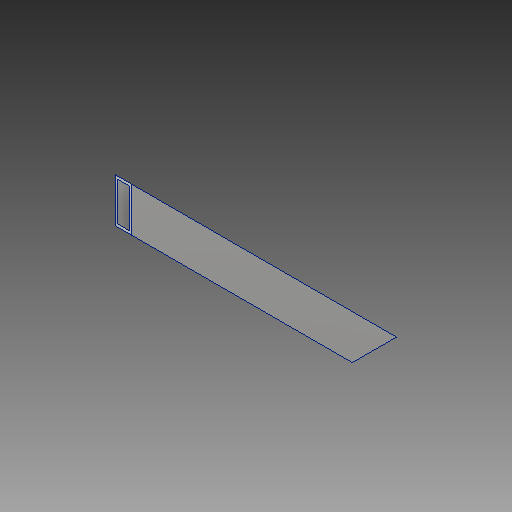
# Autodesk Inventor part: liftanglebar
Saved by Autodesk Inventor 2019 (Build 230136000, 136)
## iProperties
Created: 2019-01-13
Part Number: liftanglebar
Material: Aluminum 6061
Document SubType Name: Modeling
Designer: lebraddock
Density: 2.7 g/cm^3
Appearance: Aluminum - Flat
Mass: 670.473 g
Surface Area: 1576.79 cm^2
Volume: 248.323 cm^3
Author: lebraddock
Autodesk Inventor part; units mm, degrees
ref_plane "YZ Plane" through (0, 0, 0) normal (1, 0, 0) x (0, 1, 0)
ref_plane "XZ Plane" through (0, 0, 0) normal (0, 1, 0) x (-1, 0, 0)
ref_plane "XY Plane" through (0, 0, 0) normal (0, 0, 1) x (1, 0, 0)
sketch "Sketch1" plane through (0, 0, 0) normal (1, 0, 0) x (0, 1, 0)
  line L0 (0, -444.5) -> (444.5, 0)
  line L1 (-35.921, -408.579) -> (408.579, 35.921)
  line L2 (0, -444.5) -> (-35.921, -408.579)
  line L3 (408.579, 35.921) -> (444.5, 0)
  point P0 (0, 0)
  dimension "d1" = 444.5
  dimension "d3" = 50.8
  constraints: 8 end point, 2 parallel
  measures "d1" distance of point (0, 0) L0.start
  measures "d3" distance between parallel lines of L0 L1
extrude "Extrusion1" add sketch "Sketch1" along normal blind 25.4
sketch "Sketch2" plane through (0, 408.579, 35.921) normal (0, 0.7071, 0.7071) x (1, 0, 0)
  line L0 (0, 50.8) -> (0, 0) projected
  line L1 (0, 0) -> (25.4, 0)
  line L2 (25.4, 0) -> (25.4, 50.8)
  line L3 (25.4, 50.8) -> (0, 50.8)
  line L4 (0, 50.8) -> (0, 0)
  line L5 (3.175, 47.625) -> (22.225, 47.625)
  line L6 (22.225, 47.625) -> (22.225, 3.175)
  line L7 (22.225, 3.175) -> (3.175, 3.175)
  line L8 (3.175, 3.175) -> (3.175, 47.625)
  point P0 (0, -263.509)
  dimension "d6" = 3.175
  constraints: 16 end point, 4 parallel, 2 perpendicular, 1 horizontal, 3 other
  measures "d6" distance between parallel lines of L3 L5
extrude "Extrusion2" cut sketch "Sketch2" against normal blind 762 contours L5 L6 L7 L8
sketch "Sketch3" plane through (25.4, 0, 0) normal (1, 0, 0) x (0, 0, -1)
  line L0 (444.5, 0) -> (0, 444.5) projected
  line L1 (0, 444.5) -> (0, 339.9202)
  line L2 (0, 339.9202) -> (302.3662, 0)
  line L3 (302.3662, 0) -> (653.5481, 0)
  line L4 (653.5481, 0) -> (477.9571, -156.1918)
  line L5 (477.9571, -156.1918) -> (43.0071, -156.1918)
  line L6 (43.0071, -156.1918) -> (-176.0789, 222.25)
  line L7 (-176.0789, 222.25) -> (-134.1948, 471.4919)
  line L8 (-134.1948, 471.4919) -> (0, 494.0448)
  line L9 (0, 494.0448) -> (0, 444.5)
  point P0 (0, 0)
  constraints: 18 end point, 2 perpendicular, 1 collinear, 1 parallel, 1 point on line, 1 vertical
extrude "Extrusion3" cut sketch "Sketch3" against normal blind 25.4 contours L3 L4 L5 L6 L7 L8 L9 L1 L2
sketch "Sketch4" plane through (25.4, 0, 0) normal (1, 0, 0) x (0, 0, -1)
  line L0 (0, 0) -> (12.7, 0)
  line L1 (12.7, 0) -> (12.7, 805.7013)
  line L2 (12.7, 805.7013) -> (-196.8353, 855.7921)
  line L3 (-196.8353, 855.7921) -> (-242.5704, 324.3941)
  line L4 (-242.5704, 324.3941) -> (0, 0)
  dimension "d11" = 12.7
  constraints: 10 end point, 1 horizontal, 1 perpendicular
  measures "d11" distance of L0.start L0.end
extrude "Extrusion4" cut sketch "Sketch4" against normal blind 25.4
body "Solid1"
